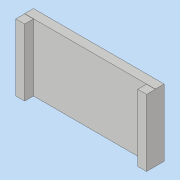
# Autodesk Inventor part: BatteryBalanceConnectorCover
Saved by Autodesk Inventor 2017 (Build 210142000, 142)
## iProperties
Created: 2019-07-16
Part Number: BatteryBalanceConnectorCover
Material: Generic
Document SubType Name: Modeling
Designer: techn
Density: 1 g/cm^3
Appearance: Default
Author: techn
Autodesk Inventor part; units mm, degrees
ref_plane "YZ Plane" through (0, 0, 0) normal (1, 0, 0) x (0, 1, 0)
ref_plane "XZ Plane" through (0, 0, 0) normal (0, 1, 0) x (-1, 0, 0)
ref_plane "XY Plane" through (0, 0, 0) normal (0, 0, 1) x (1, 0, 0)
sketch "Sketch1" plane through (0, 0, 0) normal (0, 0, 1) x (1, 0, 0)
  line L0 (0, 0) -> (18.8468, 0)
  line L1 (18.8468, 0) -> (18.8468, 9.652)
  line L2 (18.8468, 9.652) -> (0, 9.652)
  line L3 (0, 9.652) -> (0, 0)
  dimension "d0" = 18.8468
  dimension "d1" = 9.652
  constraints: 8 end point, 2 parallel, 1 horizontal, 1 perpendicular
  measures "d0" distance of L2.end L1.end
  measures "d1" distance of L1.end L0.end
extrude "Extrusion1" add sketch "Sketch1" along normal blind 1.27
sketch "Sketch2" plane through (0, 0, 1.27) normal (0, 0, 1) x (1, 0, 0)
  line L0 (0, 0) -> (18.8468, 0) projected
  line L1 (0, 0) -> (1.27, 0)
  line L2 (1.27, 0) -> (1.27, 9.6275)
  line L3 (1.27, 9.6275) -> (0, 9.6275)
  line L4 (0, 9.6275) -> (0, 0)
  line L5 (18.8468, 0) -> (17.5768, 0)
  line L6 (17.5768, 0) -> (17.5768, 9.6275)
  line L7 (17.5768, 9.6275) -> (18.8468, 9.6275)
  line L8 (18.8468, 9.6275) -> (18.8468, 0)
  dimension "d4" = 1.27
  constraints: 16 end point, 4 parallel, 2 horizontal, 2 perpendicular, 1 collinear, 1 point on line
  measures "d4" distance of L2.end L3.end
extrude "Extrusion2" add sketch "Sketch2" along normal blind 1.27
body "Solid1"
